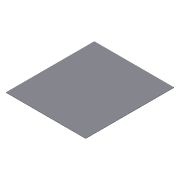
# Autodesk Inventor part: HousingCage_FloorGrid
Saved by Autodesk Inventor 2016 (Build 200138000, 138)
## iProperties
Created: 2012-11-26
Part Number: HousingCage_FloorGrid
Material: Stainless Steel
Document SubType Name: Modeling
Designer: Neef
Mass: 8475.95 g
Surface Area: 7064.75 cm^2
Volume: 1049 cm^3
Density: 8.08 g/cm^3
Appearance: Steel
Author: Neef
Autodesk Inventor part; units mm, degrees
ref_plane "YZ Plane" through (0, 0, 0) normal (1, 0, 0) x (0, 1, 0)
ref_plane "XZ Plane" through (0, 0, 0) normal (0, 1, 0) x (-1, 0, 0)
ref_plane "XY Plane" through (0, 0, 0) normal (0, 0, 1) x (1, 0, 0)
sketch "Skizze1" plane through (0, 0, 0) normal (0, 0, 1) x (1, 0, 0)
  line L0 (-301.5, -350) -> (301.5, -350)
  line L1 (301.5, -350) -> (301.5, 350)
  line L2 (301.5, 350) -> (-301.5, 350)
  line L3 (-301.5, 350) -> (-301.5, -350)
  line L4 (0, 490) -> (0, -490) projected
  line L5 (-422.1, 0) -> (422.1, 0) projected
  point P0 (0, 0)
  point P1 (-301.5, 0)
  point P2 (0, -350)
  dimension "d0" = 700
  dimension "d1" = 603
  constraints: 8 end point, 2 midpoint, 2 parallel, 2 point on line, 1 horizontal, 1 perpendicular
  measures "d0" distance of L2.end L0.start
  measures "d1" distance of L0.start L0.end
extrude "Extrusion1" add sketch "Skizze1" along normal blind 3
